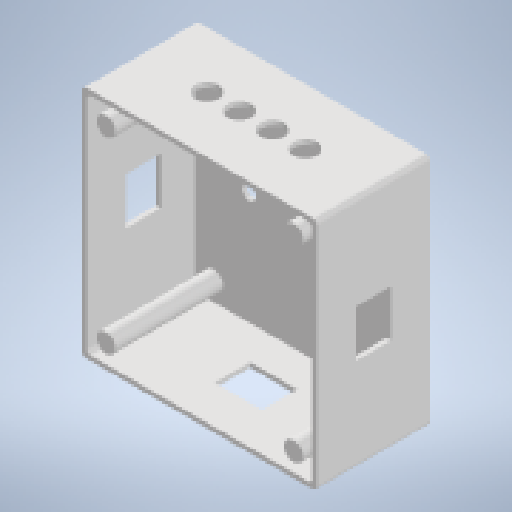
# Autodesk Inventor part: Base
Saved by Autodesk Inventor 2024 (Build 280153000, 153)
## iProperties
Created: 2023-05-04
Part Number: Base
Material: Generic
Document SubType Name: Modeling
Designer: cocqu
Density: 1 g/cm^3
Appearance: Default
Author: cocqu
Autodesk Inventor part; units mm, degrees
ref_plane "YZ Plane" through (0, 0, 0) normal (1, 0, 0) x (0, 1, 0)
ref_plane "XZ Plane" through (0, 0, 0) normal (0, 1, 0) x (-1, 0, 0)
ref_plane "XY Plane" through (0, 0, 0) normal (0, 0, 1) x (1, 0, 0)
sketch "Sketch1" plane through (0, 0, 0) normal (0, 0, 1) x (1, 0, 0)
  line L0 (-50, -50) -> (50, -50)
  line L1 (50, -50) -> (50, 50)
  line L2 (50, 50) -> (-50, 50)
  line L3 (-50, 50) -> (-50, -50)
  line L4 (-50, -50) -> (50, 50) construction
  line L5 (50, -50) -> (-50, 50) construction
  point P0 (0, 0)
  dimension "Base_Width" = 100
  dimension "Base_Length" = 100
  constraints: 12 end point, 2 midpoint, 2 parallel, 1 horizontal, 1 perpendicular
  measures "Base_Width" distance of L1.end L2.end
  measures "Base_Length" distance of L0.end L1.end
extrude "BaseBottom" add sketch "Sketch1" along normal blind 2
sketch "Sketch9" plane through (0, 0, 2) normal (0, 0, 1) x (1, 0, 0)
  line L0 (50, 50) -> (-50, 50) projected
  line L1 (0, 50) -> (0, -50) construction
  line L2 (-50, -50) -> (50, -50) projected
  circle A0 centre (-25, 0) radius 3
  circle A1 centre (25, 0) radius 3
  point P0 (0, 0)
  point P1 (0, 0)
  dimension "WallMount_Hole_Diameter" = 6
  dimension "WallMount_Hole_XPosition" = 25
  dimension "WallMount_Hole_YPosition" = 0
  constraints: 3 midpoint, 2 centre point, 2 end point, 1 symmetric about line, 1 other
  measures "WallMount_Hole_Diameter" diameter of A0
  measures "WallMount_Hole_XPosition" distance of point (0, 0) A0.centre
  measures "WallMount_Hole_YPosition" vertical distance of point (0, 0) A0.centre
extrude "WallMountHoles" [suppressed]
sketch "Sketch3" plane through (0, 0, 2) normal (0, 0, 1) x (1, 0, 0)
  line L0 (50, -50) -> (50, 50) projected
  line L1 (-50, -50) -> (50, -50)
  line L2 (50, -50) -> (50, 50)
  line L3 (50, 50) -> (-50, 50)
  line L4 (-50, 50) -> (-50, -50)
  line L5 (-50, -50) -> (50, 50) construction
  line L6 (50, -50) -> (-50, 50) construction
  line L7 (-48, 48) -> (48, 48)
  line L8 (48, 48) -> (48, -48)
  line L9 (48, -48) -> (-48, -48)
  line L10 (-48, -48) -> (-48, 48)
  point P0 (0, 0)
  point P1 (50, -50)
  dimension "Base_Wall_Thickness" = 2
  constraints: 20 end point, 4 parallel, 2 midpoint, 2 perpendicular, 1 horizontal, 3 other
  measures "Base_Wall_Thickness" distance between parallel lines of L3 L7
extrude "BaseWalls" add sketch "Sketch3" along normal blind 46
sketch "Sketch4" plane through (-50, -50, 0) normal (0, -1, 0) x (1, 0, 0)
  line L0 (40, 16.5) -> (60, 16.5)
  line L1 (60, 16.5) -> (60, 31.5)
  line L2 (60, 31.5) -> (40, 31.5)
  line L3 (40, 31.5) -> (40, 16.5)
  line L4 (40, 16.5) -> (60, 31.5) construction
  line L5 (60, 16.5) -> (40, 31.5) construction
  line L6 (50, 0) -> (50, 48) construction
  line L7 (2, 48) -> (98, 48) projected
  point P0 (50, 24)
  dimension "BatteryConnector_Hole_Width" = 20
  dimension "BatteryConnector_Hole_Height" = 15
  constraints: 14 end point, 4 midpoint, 2 parallel, 1 horizontal, 1 perpendicular
  measures "BatteryConnector_Hole_Width" distance of L1.end L2.end
  measures "BatteryConnector_Hole_Height" distance of L0.end L1.end
extrude "BatteryConnectorHole" cut sketch "Sketch4" against normal up to surface (2 mm away)
sketch "Sketch5" plane through (50, -50, 0) normal (1, 0, 0) x (0, 0, -1)
  line L0 (0, 50) -> (-48, 50) construction
  line L1 (-48, 2) -> (-48, 98) projected
  line L2 (-16.5, 40) -> (-31.5, 40)
  line L3 (-31.5, 40) -> (-31.5, 60)
  line L4 (-31.5, 60) -> (-16.5, 60)
  line L5 (-16.5, 60) -> (-16.5, 40)
  line L6 (-16.5, 40) -> (-31.5, 60) construction
  line L7 (-31.5, 40) -> (-16.5, 60) construction
  point P0 (-24, 50)
  dimension "GridConnector_Hole_Width" = 20
  dimension "GridConnector_Hole_Height" = 15
  constraints: 14 end point, 4 midpoint, 2 parallel, 1 horizontal, 1 perpendicular
  measures "GridConnector_Hole_Width" distance of L2.end L3.end
  measures "GridConnector_Hole_Height" distance of L3.end L4.end
extrude "GridConnectorHole" cut sketch "Sketch5" against normal up to surface (2 mm away)
sketch "Sketch6" plane through (-50, -50, 0) normal (-1, 0, 0) x (0, 0, 1)
  line L0 (0, 50) -> (48, 50) construction
  line L1 (48, 2) -> (48, 98) projected
  line L2 (16.5, 60) -> (31.5, 60)
  line L3 (31.5, 60) -> (31.5, 40)
  line L4 (31.5, 40) -> (16.5, 40)
  line L5 (16.5, 40) -> (16.5, 60)
  line L6 (16.5, 60) -> (31.5, 40) construction
  line L7 (31.5, 60) -> (16.5, 40) construction
  point P0 (24, 50)
  dimension "DeviceConnector_Hole_Width" = 20
  dimension "DeviceConnector_Hole_Height" = 15
  constraints: 14 end point, 4 midpoint, 2 parallel, 1 horizontal, 1 perpendicular
  measures "DeviceConnector_Hole_Width" distance of L2.end L3.end
  measures "DeviceConnector_Hole_Height" distance of L3.end L4.end
extrude "DeviceConnectorHole" cut sketch "Sketch6" against normal up to surface (2 mm away)
sketch "Sketch8" plane through (-50, 50, 0) normal (0, 1, 0) x (1, 0, 0)
  line L0 (0, 0) -> (0, -48) projected
  line L1 (0, -24) -> (100, -24) construction
  line L2 (100, 0) -> (100, -48) projected
  circle A0 centre (29, -24) radius 5
  circle A1 centre (43, -24) radius 5
  circle A2 centre (57, -24) radius 5
  circle A3 centre (71, -24) radius 5
  point P0 (50, 0)
  point P1 (50, -24)
  dimension "Distance_Between_Buttons" = 14
  dimension "Button_Hole_Diameter" = 10
  dimension "Center_Buttons" = 21
  constraints: 4 centre point, 3 midpoint, 2 end point, 1 horizontal, 1 point on line, 6 other
  measures "Distance_Between_Buttons" distance of A0.centre A1.centre
  measures "Button_Hole_Diameter" diameter of A0
  measures "Center_Buttons" distance of point (50, -24) A0.centre
extrude "ButtonHoles" cut sketch "Sketch8" against normal up to surface (2 mm away)
fillet "BaseCorners" radius 2 8 edges at (-50, 50, 24) (50, 50, 24) (50, -50, 24) (-50, -50, 24) (-48, -48, 25) (-48, 48, 25) (48, 48, 25) (48, -48, 25)
sketch "Sketch11" plane through (0, 0, 2) normal (0, 0, 1) x (1, 0, 0)
  circle A0 centre (-40, 40) radius 4
  line L0 (48, 50) -> (-48, 50) projected
  line L1 (-50, 48) -> (-50, -48) projected
  line L2 (0, 0) -> (0, 50) construction
  line L3 (0, 0) -> (-50, 0) construction
  circle A1 centre (40, 40) radius 4
  circle A2 centre (-40, -40) radius 4
  circle A3 centre (40, -40) radius 4
  dimension "d64" = 8
  dimension "d65" = 10
  dimension "d66" = 10
  constraints: 4 centre point, 4 end point, 3 symmetric about line, 2 midpoint, 3 other
  measures "d64" diameter of A0
  measures "d65" distance from line of L0 A0.centre
  measures "d66" distance from line of L1 A0.centre
extrude "Extrusion11" add sketch "Sketch11" along normal blind 46
sketch "Sketch12" plane through (-40, 40, 48) normal (0, 0, 1) x (1, 0, 0)
  circle A0 centre (80, -80) radius 4 projected
  circle A1 centre (80, -80) radius 1.65
  circle A2 centre (0, 0) radius 1.65
  circle A3 centre (80, 0) radius 1.65
  circle A4 centre (0, -80) radius 1.65
  circle A5 centre (0, -80) radius 4 projected
  circle A6 centre (0, 0) radius 4 projected
  circle A7 centre (80, 0) radius 4 projected
  point P0 (40, -40)
  dimension "d69" = 3.3
  dimension "d70" = 3.3
  dimension "d71" = 3.3
  dimension "d72" = 3.3
  dimension "d73" = 0
  dimension "d74" = 0
  dimension "d75" = 0
  dimension "d76" = 0
  dimension "d77" = 0
  dimension "d78" = 0
  constraints: 4 centre point, 1 coincident
  measures "d69" diameter of A1
  measures "d70" diameter of A2
  measures "d71" diameter of A3
  measures "d72" diameter of A4
  measures "d73" distance of A5.centre A4.centre
  measures "d74" distance of A5.centre A4.centre
  measures "d75" distance of A6.centre A2.centre
  measures "d76" distance of A6.centre A2.centre
  measures "d77" distance of A7.centre A3.centre
  measures "d78" distance of A7.centre A3.centre
extrude "Extrusion12" cut sketch "Sketch12" against normal blind 20 contours A1 | A2 | A3 | A4
fillet "Fillet2" radius 0.5 4 edges at (16, 50, 24) (2, 50, 24) (-12, 50, 24) (-26, 50, 24)
fillet "Fillet3" radius 4 12 edges at (49, 10, 31.5) (49, 10, 16.5) (49, -10, 31.5) (49, -10, 16.5) (-10, -49, 16.5) (10, -49, 16.5) (-10, -49, 31.5) (10, -49, 31.5) (-49, 10, 16.5) (-49, 10, 31.5) (-49, -10, 16.5) (-49, -10, 31.5)
equation "\"Base_Width\" = PCB_Width + 2 * Offset"
equation "\"Base_Length\" = PCB_Length + 2 * Offset"
equation "\"Base_Bottom_Thickness\" = Wall_Thickness"
equation "\"WallMount_Hole_XPosition\" = 0.25 * Base_Width"
equation "\"Base_Wall_Thickness\" = Wall_Thickness"
equation "\"Base_Height\" = Offset + PCB_Height - 2 * Wall_Thickness"
equation "\"d15\" = PCB_Height + Offset"
equation "\"Distance_Between_Buttons\" = Button_Diameter + Button_Distance_Between"
equation "\"Button_Hole_Diameter\" = Button_Diameter"
equation "\"d37\" = Wall_Thickness"
equation "\"d67\" = Offset + PCB_Height - 2 * Wall_Thickness"
equation "\"PCB_Height\" = 40"
equation "\"Wall_Thickness\" = 2"
equation "\"Offset\" = 10"
equation "\"Button_Distance_Between\" = 4"
equation "\"Button_Diameter\" = 10"
equation "\"PCB_Width\" = 80"
equation "\"PCB_Length\" = 80"
body "Solid1"
